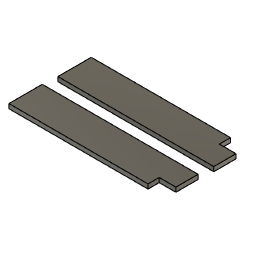
Abdeckung Profielschiene unten (Autodesk Fusion 360 design; units mm, degrees)
Autodesk Fusion 360 part; units mm, degrees
sketch "Skizze1" plane through (0, 0, 0) normal (0, 0, 1) x (1, 0, 0)
  line L0 (10, 5) -> (290, 5)
  line L1 (290, 5) -> (290, 35)
  line L2 (290, 35) -> (10, 35)
  line L3 (10, 35) -> (10, 5)
  dimension "d1" = 280
  dimension "d2" = 30
  constraint horizontal L0
  constraint vertical L1
  constraint horizontal L2
  constraint vertical L3
  measures "d1" distance of L0.start L0.end
  measures "d2" distance of L0.start L2.end
extrude "Extrusion1" add sketch "Skizze1" along normal blind 1 makes body 1
sketch "Skizze2" plane through (0, 0, 1) normal (0, 0, 1) x (-1, 0, 0)
  line L0 (-10, -35) -> (-10, -5)
  line L1 (-10, -5) -> (-290, -5)
  line L2 (-290, -5) -> (-290, -35)
  line L3 (-290, -35) -> (-10, -35)
  line L4 (-10, -35) -> (-25, -35)
  line L5 (-25, -35) -> (-25, -25)
  line L6 (-25, -25) -> (-10, -25)
  line L7 (-10, -25) -> (-10, -35)
  line L8 (-290, -35) -> (-275, -35)
  line L9 (-275, -35) -> (-275, -25)
  line L10 (-275, -25) -> (-290, -25)
  line L11 (-290, -25) -> (-290, -35)
  dimension "d5" = 10
  dimension "d6" = 10
  dimension "d7" = 15
  dimension "d8" = 15
  constraint horizontal L4
  constraint vertical L5
  constraint horizontal L6
  constraint vertical L7
  constraint coincident L0.start L3.end
  constraint horizontal L8
  constraint vertical L9
  constraint horizontal L10
  constraint vertical L11
  constraint coincident L2.end L3.start
  measures "d5" distance of L8.end L9.end
  measures "d6" distance of L4.end L5.end
  measures "d7" distance of L0.start L4.end
  measures "d8" distance of L2.end L8.end
extrude "Extrusion2" cut sketch "Skizze2" against normal blind 15 contours L0 L3 L4 L5 L6 L7 | L2 L3 L8 L9 L10 L11 bodies 1
sketch "Skizze3" plane through (0, 0, 1) normal (0, 0, 1) x (-1, 0, 0)
  line L0 (-25, -25) -> (-10, -25)
  line L1 (-10, -25) -> (-10, -5)
  line L2 (-10, -5) -> (-290, -5)
  line L3 (-290, -5) -> (-290, -25)
  line L4 (-290, -25) -> (-275, -25)
  line L5 (-275, -25) -> (-275, -35)
  line L6 (-275, -35) -> (-25, -35)
  line L7 (-25, -35) -> (-25, -25)
  line L8 (-10, -2.919) -> (-150, -2.919)
  line L9 (-150, -2.919) -> (-150, -38)
  line L10 (-150, -38) -> (-10, -38)
  line L11 (-10, -38) -> (-10, -2.919)
  dimension "d11" = 140
  constraint horizontal L8
  constraint vertical L9
  constraint horizontal L10
  constraint vertical L11
  constraint coincident L1 L8.start
  measures "d11" distance of L8.start L8.end
extrude "Extrusion3" cut sketch "Skizze3" against normal blind 20 contours L0 L1 L2 L6 L7 L9 L11 | L0 L6 L7 L9 L10 L11 | L2 L8 L9 L11 bodies 1
sketch "Skizze4" plane through (0, 0, 1) normal (0, 0, 1) x (-1, 0, 0)
  line L0 (-150, -35) -> (-150, -5)
  line L1 (-150, -5) -> (-290, -5)
  line L2 (-290, -5) -> (-290, -25)
  line L3 (-290, -25) -> (-275, -25)
  line L4 (-275, -25) -> (-275, -35)
  line L5 (-275, -35) -> (-150, -35)
  line L6 (-150, 0) -> (-290, 0)
  line L7 (-290, 0) -> (-290, 2)
  line L8 (-290, 2) -> (-150, 2)
  line L9 (-150, 2) -> (-150, 0)
  line L10 (-275, 29) -> (-275, 39)
  line L11 (-290, 29) -> (-275, 29)
  line L12 (-275, 39) -> (-150, 39)
  line L13 (-150, 39) -> (-150, 9)
  line L14 (-150, 9) -> (-290, 9)
  line L15 (-290, 9) -> (-290, 29)
  constraint horizontal L6
  constraint vertical L7
  constraint horizontal L8
  constraint vertical L9
  constraint symmetric L0.start L8 L12.end
  constraint symmetric L0.end L8 L13.end
  constraint symmetric L1.end L8 L14.end
  constraint symmetric L2.end L8 L11.start
  constraint symmetric L3.end L8 L10.start
  constraint symmetric L4.end L8 L10.end
extrude "Extrusion4" add sketch "Skizze4" along normal blind 4 separate body contours L10 L11 L12 L13 L14 L15 makes body 2
extrude "Extrusion5" add 1 faces at (191.6667, 21.6667, 1) along direction (0, 0, 1) blind 3 on bodies 1 bodies 1
